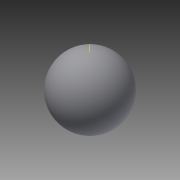
# Autodesk Inventor part: Ball Bearing 3- 16  in
Saved by Autodesk Inventor 2013 (Build 170138000, 138)
## iProperties
Created: 2013-06-06
Part Number: Ball Bearing 3- 16  in
Material: Generic
Document SubType Name: Modeling
Designer: mvarma
Density: 1 g/cm^3
Author: mvarma
Autodesk Inventor part; units mm, degrees
ref_plane "XZ Plane" through (0, 0, 0) normal (0, 1, 0) x (-1, 0, 0)
ref_plane "XY Plane" through (0, 0, 0) normal (0, 0, 1) x (1, 0, 0)
sketch "Sketch1" plane through (0, 0, 0) normal (0, 0, 1) x (1, 0, 0)
  arc A0 (-2.3812, 0) -> (2.3813, 0) centre (0, 0) ccw
  line L0 (-2.3812, 0) -> (2.3813, 0)
  dimension "d0" = 4.7625
  dimension "d1" = 4.7625
  constraints: 2 end point, 2 point on circle, 1 centre point, 1 coincident, 1 horizontal
  measures "d0" diameter of A0
  measures "d1" distance of L0.start L0.end
revolve "Revolution1" add sketch "Sketch1" angle 360 about axis through (-2.3812, 0, 0) along (1, 0, 0)
equation "\"d1\" = d0"
body "Solid1"
